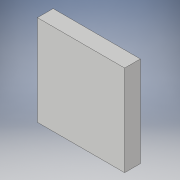
# Autodesk Inventor part: LpmsB2_moldes_inventor_mesh
Saved by Autodesk Inventor 2019.4 (Build 234330000, 330)
## iProperties
Created: 2021-05-02
Part Number: LpmsB2_moldes_inventor_mesh
Material: Generic
Document SubType Name: Modeling
Designer: mx19
Density: 1 g/cm^3
Appearance: Default
Author: mx19
Autodesk Inventor part; units mm, degrees
ref_plane "YZ Plane" through (0, 0, 0) normal (1, 0, 0) x (0, 1, 0)
ref_plane "XZ Plane" through (0, 0, 0) normal (0, 1, 0) x (-1, 0, 0)
ref_plane "XY Plane" through (0, 0, 0) normal (0, 0, 1) x (1, 0, 0)
sketch "Sketch1" plane through (-1958.9195, -63.7501, 156.7315) normal (0, 0, 1) x (1, 0, 0)
  line L0 (-934.3699, 1296.4339) -> (1108.8849, 1296.4339)
  line L1 (1108.8849, 1296.4339) -> (1108.8849, -826.7744)
  line L2 (1108.8849, -826.7744) -> (-934.3699, -826.7744)
  line L3 (-934.3699, -826.7744) -> (-934.3699, 1296.4339)
  point P0 (1958.9195, 63.7501)
  constraints: 8 end point, 2 parallel, 1 horizontal, 1 perpendicular
extrude "Extrusion1" add sketch "Sketch1" along normal blind 203.2 and the other way blind 165.1
body "Solid1"
